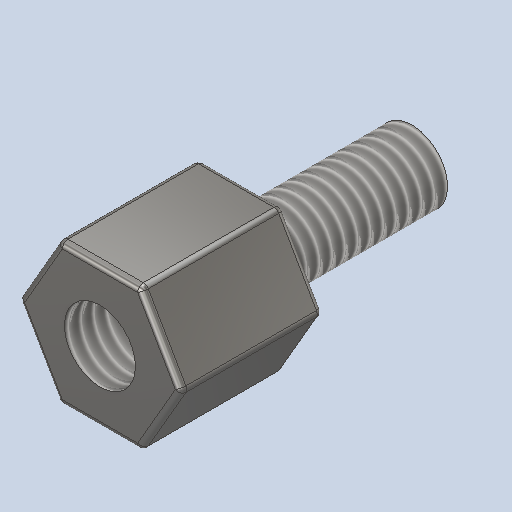
# Autodesk Inventor part: M2.5 Hex Spacer 5mm
Saved by Autodesk Inventor 2023 (Build 270158000, 158)
## iProperties
Created: 2020-05-05
Part Number: M2.5 Hex Spacer 5mm
Material: Stainless Steel
Document SubType Name: Modeling
Designer: Mike Angus
Density: 8 g/cm^3
Appearance: Semi-Polished
m3hs_bodyLength: 5,000 mm
m3hs_holeDepth: 3,000 mm
m3hs_studLength: 6,000 mm
Author: Mike Angus
Autodesk Inventor part; units mm, degrees
ref_plane "YZ Plane" through (0, 0, 0) normal (1, 0, 0) x (0, 1, 0)
ref_plane "XZ Plane" through (0, 0, 0) normal (0, 1, 0) x (-1, 0, 0)
ref_plane "XY Plane" through (0, 0, 0) normal (0, 0, 1) x (1, 0, 0)
sketch "Sketch1" plane through (0, 0, 0) normal (0, 0, 1) x (1, 0, 0)
  line L0 (1.4434, -2.5) -> (-1.4434, -2.5)
  line L1 (-1.4434, -2.5) -> (-2.8868, 0)
  line L2 (-2.8868, 0) -> (-1.4434, 2.5)
  line L3 (-1.4434, 2.5) -> (1.4434, 2.5)
  line L4 (1.4434, 2.5) -> (2.8868, 0)
  line L5 (2.8868, 0) -> (1.4434, -2.5)
  point P0 (0, 0)
  point P1 (0, 0)
  dimension "d0" = 5
  constraints: 12 end point, 1 coincident, 1 horizontal, 13 other
  measures "d0" distance between parallel lines of L3 L0
extrude "Extrusion1" add sketch "Sketch1" against normal blind 5
sketch "Sketch2" plane through (0, 0, 0) normal (0, 0, 1) x (1, 0, 0)
  circle A0 centre (0, 0) radius 1.25
  dimension "d3" = 2.5
  constraints: 1 centre point, 1 coincident
  measures "d3" diameter of A0
extrude "Extrusion2" cut sketch "Sketch2" against normal blind 3
sketch "Sketch3" plane through (0, 0, -5) normal (0, 0, -1) x (-1, 0, 0)
  circle A0 centre (0, 0) radius 1.25
  dimension "d6" = 2.5
  constraints: 1 centre point, 1 coincident
  measures "d6" diameter of A0
extrude "Extrusion3" add sketch "Sketch3" along normal blind 6
thread "Thread1" size "M2.5x0.45" class "6g" standard "ISO Metric profile" full length
thread "Thread2" size "M2.5x0.45" class "6H" standard "ISO Metric profile" full length
fillet "Fillet1" radius 0.2 12 edges at (0, -2.5, -5) (-2.1651, -1.25, -5) (-2.1651, 1.25, -5) (0, 2.5, -5) (2.1651, 1.25, -5) (2.1651, -1.25, -5) (0, -2.5, 0) (2.1651, -1.25, 0) (2.1651, 1.25, 0) (0, 2.5, 0) (-2.1651, 1.25, 0) (-2.1651, -1.25, 0)
fillet "Fillet1" radius 0.2 6 edges at (-2.8868, 0, -2.5) (-1.4434, 2.5, -2.5) (1.4434, 2.5, -2.5) (2.8868, 0, -2.5) (1.4434, -2.5, -2.5) (-1.4434, -2.5, -2.5)
equation "\"d0\" = m3hs_hexDiam"
equation "\"d1\" = m3hs_bodyLength"
equation "\"d3\" = m3hs_threadDiam"
equation "\"d4\" = m3hs_holeDepth"
equation "\"d6\" = m3hs_threadDiam"
equation "\"d7\" = m3hs_studLength"
equation "\"d13\" = m3hs_rounding"
equation "\"m3hs_hexDiam\" = 5"
equation "\"m3hs_bodyLength\" = 5"
equation "\"m3hs_holeDepth\" = 3"
equation "\"m3hs_studLength\" = 6"
equation "\"m3hs_rounding\" = 0.2"
equation "\"m3hs_threadDiam\" = 2.5"
body "Solid1"
